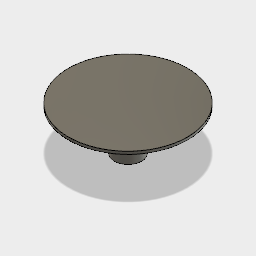
socle 1 (Autodesk Fusion 360 design; units mm, degrees)
Autodesk Fusion 360 part; units mm, degrees
sketch "Sketch1" plane through (0, 0, 0) normal (0, 0, 1) x (1, 0, 0)
  line L0 (0, 48) -> (0, 0)
  line L1 (0, 0) -> (15, 0)
  line L2 (15, 0) -> (15, 30)
  line L3 (30, 45) -> (65, 45)
  line L4 (65, 45) -> (65, 48)
  line L5 (65, 48) -> (0, 48)
  arc A0 (30, 45) -> (15, 30) centre (30, 30) ccw
  arc A1 (30, 45) -> (15, 30) centre (30, 30) ccw
  dimension "d1" = 15
  dimension "d2" = 15
  dimension "d3" = 65
  dimension "d4" = 3
  dimension "d6" = 30
  measures "d1" radius of A0
  measures "d2" distance of L0.end L1.end
  measures "d3" distance of L0.start L4.end
  measures "d4" distance of L3.end L4.end
  measures "d6" distance of L1.end L2.end
revolve "Revolve1" add sketch "Sketch1" angle 360 about axis through (0, 48, 0) along (0, -1, 0)
hole "Hole1" at (0, 0, 0) direction (0, 1, 0) diameter 26 depth 30 tip angle 150
